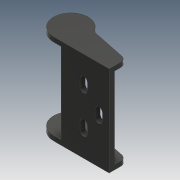
# Autodesk Inventor part: carrier-end
Saved by Autodesk Inventor 2017 (Build 210142000, 142)
## iProperties
Created: 2018-06-20
Part Number: carrier-end
Material: ABS Plastic
Document SubType Name: Modeling
Designer: Luiz Gustavo
Density: 1.06 g/cm^3
Appearance: Smooth - Black
Author: Luiz Gustavo
Autodesk Inventor part; units mm, degrees
ref_plane "YZ Plane" through (0, 0, 0) normal (1, 0, 0) x (0, 1, 0)
ref_plane "XZ Plane" through (0, 0, 0) normal (0, 1, 0) x (-1, 0, 0)
ref_plane "XY Plane" through (0, 0, 0) normal (0, 0, 1) x (1, 0, 0)
sketch "Sketch1" plane through (0, 0, 0) normal (0, 0, 1) x (1, 0, 0)
  circle A0 centre (0, 0) radius 11.5
  line L0 (5, -11.5) -> (37, -11.5)
  line L1 (37, -11.5) -> (37, -8)
  line L2 (37, -8) -> (5, -8)
  line L3 (5, -8) -> (5, -11.5)
  line L4 (37, -8) -> (37, -0.5)
  line L5 (37, -0.5) -> (10.3562, 5)
  line L6 (0, 0) -> (0, -11.5) construction
  line L7 (0, -11.5) -> (5, -11.5)
  dimension "d0" = 23
  dimension "d2" = 3.5
  dimension "d3" = 11
  dimension "d4" = 5
  dimension "d5" = 5
  dimension "d6" = 37
  constraints: 16 end point, 3 vertical, 2 horizontal, 2 perpendicular, 2 point on circle, 1 centre point, 1 coincident
  measures "d0" diameter of A0
  measures "d2" distance of L0.end L1.end
  measures "d3" distance of L0.end L4.end
  measures "d4" vertical distance of point (0, 0) L5.end
  measures "d5" distance between parallel lines of L6 L3
  measures "d6" distance between parallel lines of L6 L1
extrude "Extrusion1" add sketch "Sketch1" along normal mid plane 60
extrude "Extrusion2" cut sketch "Sketch1" along normal mid plane 54 contours A0 L2 L3 | A0 L5 L4 L2 | A0 L3 L7 picked at (-2.9713, 3.3704)
sketch "Sketch2" plane through (0, 0, 0) normal (0, 1, 0) x (-1, 0, 0)
  line L0 (0, 0) -> (-30, 0) construction
  arc A0 (-27.5, -2.5) -> (-32.5, -2.5) centre (-30, -2.5) ccw construction
  arc A1 (-32.5, 2.5) -> (-27.5, 2.5) centre (-30, 2.5) ccw construction
  line L1 (-32.5, -2.5) -> (-32.5, 2.5)
  line L2 (-27.5, -2.5) -> (-27.5, 2.5)
  line L3 (-30, -2.5) -> (-30, 2.5) construction
  arc A2 (-32.5, -2.5) -> (-27.5, -2.5) centre (-30, -2.5) ccw
  arc A3 (-27.5, 2.5) -> (-32.5, 2.5) centre (-30, 2.5) ccw
  line L4 (-22.5, -15) -> (-22.5, -10)
  line L5 (-17.5, -15) -> (-17.5, -10)
  arc A4 (-22.5, -15) -> (-17.5, -15) centre (-20, -15) ccw
  arc A5 (-17.5, -10) -> (-22.5, -10) centre (-20, -10) ccw
  line L6 (-20, -15) -> (-20, -10) construction
  arc A6 (-17.5, 15) -> (-22.5, 15) centre (-20, 15) ccw
  line L7 (-22.5, 15) -> (-22.5, 10)
  line L8 (-17.5, 15) -> (-17.5, 10)
  arc A7 (-22.5, 10) -> (-17.5, 10) centre (-20, 10) ccw
  line L9 (-20, 15) -> (-20, 10) construction
  line L10 (-17.5, -12.5) -> (-22.5, -12.5) construction
  line L11 (-17.5, 12.5) -> (-22.5, 12.5) construction
  dimension "d13" = 30
  dimension "d18" = 5
  dimension "d19" = 5
  dimension "d22" = 10
  dimension "d23" = 25
  constraints: 24 end point, 16 point on circle, 8 centre point, 8 symmetric about line, 6 vertical, 4 tangent, 3 equal radius, 3 midpoint, 1 horizontal, 1 parallel, 2 other
  measures "d13" distance of L0.end L0.start
  measures "d18" diameter of A0
  measures "d19" distance of L3.end L3.start
  measures "d22" distance from line of L0.end L6
  measures "d23" distance between parallel lines of L11 L10
extrude "Extrusion3" cut sketch "Sketch2" against normal through all
fillet "Fillet1" radius 4 4 edges at (37, -0.5, -28.5) (37, -0.5, 28.5) (10.3562, 5, -28.5) (10.3562, 5, 28.5)
body "Solid1"
